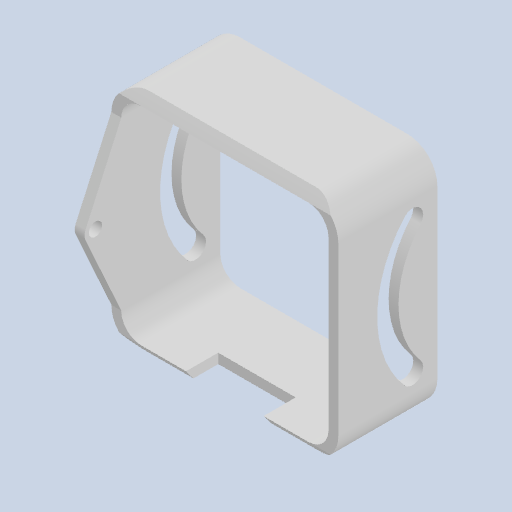
# Autodesk Inventor part: lidar_base
Saved by Autodesk Inventor 2022 (Build 260153000, 153)
## iProperties
Created: 2024-10-20
Part Number: lidar_base
Material: Типовые
Document SubType Name: Modeling
Designer: Andrey
Density: 1 g/cm^3
Appearance: По умолчанию
Author: Andrey
Autodesk Inventor part; units mm, degrees
ref_plane "YZ Plane" through (0, 0, 0) normal (1, 0, 0) x (0, 1, 0)
ref_plane "РабПлоскость1" through (-16.75, -17.4, 16.3) normal (0, 0, 1) x (1, 0, 0)
sketch "Эскиз1" plane through (0, 0, 0) normal (0, 0, 1) x (1, 0, 0)
  line L0 (-18.1779, 4.2816) -> (-18.69, 4.2816) projected
  line L1 (-18.69, 4.2816) -> (-18.69, -13.75) projected
  arc A0 (-18.69, -13.75) -> (-13.75, -18.69) centre (-13.75, -13.75) ccw projected
  line L2 (-13.75, -18.69) -> (13.75, -18.69) projected
  arc A1 (13.75, -18.69) -> (18.69, -13.75) centre (13.75, -13.75) ccw projected
  line L3 (18.69, -13.75) -> (18.69, 13.75) projected
  arc A2 (18.69, 13.75) -> (13.75, 18.69) centre (13.75, 13.75) ccw projected
  line L4 (13.75, 18.69) -> (-13.75, 18.69) projected
  arc A3 (-13.75, 18.69) -> (-18.69, 13.75) centre (-13.75, 13.75) ccw projected
  line L5 (-18.69, 13.75) -> (-18.69, 9.7184) projected
  line L6 (-18.69, 9.7184) -> (-18.1779, 9.7184) projected
  line L7 (-18.1779, 13.75) -> (-18.1779, 9.7184) projected
  arc A4 (-13.75, 18.1779) -> (-18.1779, 13.75) centre (-13.75, 13.75) ccw projected
  line L8 (13.75, 18.1779) -> (-13.75, 18.1779) projected
  arc A5 (18.1779, 13.75) -> (13.75, 18.1779) centre (13.75, 13.75) ccw projected
  line L9 (18.1779, -13.75) -> (18.1779, 13.75) projected
  arc A6 (13.75, -18.1779) -> (18.1779, -13.75) centre (13.75, -13.75) ccw projected
  line L10 (-13.75, -18.1779) -> (13.75, -18.1779) projected
  arc A7 (-18.1779, -13.75) -> (-13.75, -18.1779) centre (-13.75, -13.75) ccw projected
  line L11 (-18.1779, 4.2816) -> (-18.1779, -13.75) projected
  line L12 (-18.1779, 4.2816) -> (-18.69, 4.2816)
  line L13 (-18.69, 4.2816) -> (-18.69, 9.7184)
  line L14 (-18.69, 9.7184) -> (-18.1779, 9.7184)
  line L15 (-18.1779, 9.7184) -> (-18.1779, 4.2816)
  line L16 (-13.75, 16.45) -> (10.2, 16.45) projected
  arc A8 (-13.75, 16.45) -> (-16.75, 13.45) centre (-13.75, 13.45) ccw projected
  line L17 (-16.75, -10.2) -> (-16.75, 13.45) projected
  arc A9 (-16.75, -10.2) -> (-15.75, -11.2) centre (-15.75, -10.2) ccw projected
  line L18 (-14.1, -11.2) -> (-15.75, -11.2) projected
  arc A10 (-11.2, -14.1) -> (-14.1, -11.2) centre (-14.1, -14.1) ccw projected
  line L19 (-11.2, -14.1) -> (-11.2, -15.75) projected
  arc A11 (-11.2, -15.75) -> (-10.2, -16.75) centre (-10.2, -15.75) ccw projected
  line L20 (-6.3858, -16.75) -> (-10.2, -16.75) projected
  arc A12 (-5.9929, -17.075) -> (-6.3858, -16.75) centre (-6.3858, -17.15) ccw projected
  arc A13 (-5.9929, -17.075) -> (-5.6, -17.4) centre (-5.6, -17) ccw projected
  line L21 (-5.6, -17.4) -> (5.6, -17.4) projected
  arc A14 (5.6, -17.4) -> (5.9929, -17.075) centre (5.6, -17) ccw projected
  arc A15 (6.3858, -16.75) -> (5.9929, -17.075) centre (6.3858, -17.15) ccw projected
  line L22 (12.1982, -16.75) -> (6.3858, -16.75) projected
  arc A16 (12.1982, -16.75) -> (13.1981, -15.7356) centre (12.1982, -15.75) ccw projected
  arc A17 (15.7351, -13.198) -> (13.1981, -15.7356) centre (15.6978, -15.6978) ccw projected
  arc A18 (15.7351, -13.198) -> (16.75, -12.1982) centre (15.75, -12.1982) ccw projected
  line L23 (16.75, -12.1982) -> (16.75, 10.2) projected
  arc A19 (16.75, 10.2) -> (15.75, 11.2) centre (15.75, 10.2) ccw projected
  line L24 (14.1, 11.2) -> (15.75, 11.2) projected
  arc A20 (11.2, 14.1) -> (14.1, 11.2) centre (14.1, 14.1) ccw projected
  line L25 (11.2, 15.45) -> (11.2, 14.1) projected
  arc A21 (11.2, 15.45) -> (10.2, 16.45) centre (10.2, 15.45) ccw projected
  circle A22 centre (7, 14.5) radius 0.95 projected
  circle A23 centre (0, 14.6) radius 0.75 projected
  circle A24 centre (-7.5, -13.8) radius 0.95 projected
  circle A25 centre (-14.9, 2) radius 0.75 projected
  circle A26 centre (8.272, -2.7758) radius 0.5 projected
  circle A27 centre (8.6932, -0.0132) radius 0.5 projected
  circle A28 centre (8.2597, 2.7621) radius 0.5 projected
  circle A29 centre (-2.2984, 14.2551) radius 0.5 projected
  circle A30 centre (-4.5412, 14.2552) radius 0.5 projected
  circle A31 centre (13.75, -13.75) radius 3.5
  circle A32 centre (-13.75, -13.75) radius 3.5
  circle A33 centre (13.75, 13.75) radius 3.5
  circle A34 centre (-13.75, 13.75) radius 3.5
  line L26 (-17.25, 13.75) -> (-17.25, -13.75)
  line L27 (-13.75, -17.25) -> (13.75, -17.25)
  line L28 (17.25, -13.75) -> (17.25, 13.75)
  line L29 (13.75, 17.25) -> (-13.75, 17.25)
  arc A35 (13.75, -17.25) -> (17.25, -13.75) centre (13.75, -13.75) ccw
  arc A36 (-17.25, -13.75) -> (-13.75, -17.25) centre (-13.75, -13.75) ccw
  arc A37 (-13.75, 17.25) -> (-17.25, 13.75) centre (-13.75, 13.75) ccw
  arc A38 (17.25, 13.75) -> (13.75, 17.25) centre (13.75, 13.75) ccw
  line L30 (-13.75, 17.05) -> (13.75, 17.05)
  arc A39 (17.05, 13.75) -> (13.75, 17.05) centre (13.75, 13.75) ccw
  line L31 (17.05, 13.75) -> (17.05, -13.75)
  arc A40 (13.75, -17.05) -> (17.05, -13.75) centre (13.75, -13.75) ccw
  line L32 (13.75, -17.05) -> (-13.75, -17.05)
  arc A41 (-17.05, -13.75) -> (-13.75, -17.05) centre (-13.75, -13.75) ccw
  line L33 (-17.05, -13.75) -> (-17.05, 13.75)
  arc A42 (-13.75, 17.05) -> (-17.05, 13.75) centre (-13.75, 13.75) ccw
  line L34 (6.3858, -18.69) -> (-6.3858, -18.69)
  line L35 (-6.3858, -18.69) -> (-6.3858, -14.69)
  line L36 (-6.3858, -14.69) -> (6.3858, -14.69)
  line L37 (6.3858, -14.69) -> (6.3858, -18.69)
  point P0 (0, 0)
  point P1 (12.5838, -17.05)
  point P2 (5.9122, -17.25)
  point P3 (5.9985, -17.05)
  point P4 (-6.3858, -17.05)
  point P5 (6.3858, -17.05)
  point P6 (-6.3858, -18.69)
  dimension "d0" = 7
  dimension "d2" = 7
  dimension "d3" = 7
  dimension "d4" = 7
  dimension "d5" = 0.2
  dimension "d8" = 4
  constraints: 32 end point, 24 point on circle, 12 centre point, 12 tangent, 4 coincident, 4 parallel, 3 point on line, 2 concentric, 2 horizontal, 2 perpendicular, 7 other
  measures "d0" diameter of A31
  measures "d2" diameter of A32
  measures "d3" diameter of A33
  measures "d4" diameter of A34
  measures "d5" distance between parallel lines of L29 L30
  measures "d8" distance of L34.end L35.end
extrude "Выдавливание1" add sketch "Эскиз1" along normal up to surface (16.3 mm away) contours L11 A7 L10 L35 L2 A0 L1 L0 | L15 L7 A4 L8 A5 L9 A6 L10 L37 L27 A31 L28 A33 L29 A34 L26 A32 L35 A7 L11 | L0 L13 L6 L15 | L6 L5 A3 L4 A2 L3 A1 L2 L37 L10 A6 L9 A5 L8 A4 L7 | L27 A32 L32 L35 | L37 L32 A31 L27 | A32 L33 A41 L32 | A31 L32 A40 L31 | L26 A34 L33 A32 | A31 L31 A33 L28 | A34 L30 A42 L33 | A33 L31 A39 L30 | L29 A33 L30 A34
sketch "Эскиз2" plane through (0, 0, 0) normal (0, 0, -1) x (-1, 0, 0)
  line L0 (6.3858, -18.69) -> (6.3858, -17.05) projected
  line L1 (-6.3858, -17.05) -> (-6.3858, -18.69) projected
  line L2 (6.3858, -18.69) -> (-6.3858, -18.69)
  line L3 (-6.3858, -18.69) -> (-6.3858, -17.05)
  line L4 (-6.3858, -17.05) -> (6.3858, -17.05)
  line L5 (6.3858, -17.05) -> (6.3858, -18.69)
  point P0 (0, 0)
  constraints: 8 end point, 2 parallel, 1 horizontal, 1 perpendicular
extrude "Выдавливание2" add sketch "Эскиз2" against normal blind 11
sketch "Эскиз3" plane through (-18.69, -13.75, 0) normal (-1, 0, 0) x (0, 0, 1)
  circle A0 centre (-8.4, 13.75) radius 18.69 projected
  line L0 (0, 13.75) -> (16.3, 13.75)
  line L1 (16.3, 27.5) -> (16.3, 0) projected
  circle A1 centre (-8.4, 13.75) radius 14.8
  line L2 (0, 13.75) -> (16.3, 13.75)
  line L3 (0, 0) -> (0, 27.5) projected
  circle A2 centre (8.15, 13.75) radius 1.75
  circle A3 centre (-8.4, 13.75) radius 18.3
  circle A4 centre (4.0904, 24.6078) radius 1.75
  circle A5 centre (4.0904, 2.8922) radius 1.75
  line L4 (-8.4, 13.75) -> (22.7381, 2.4167) projected
  line L5 (-8.4, 13.75) -> (22.7381, 25.0833) projected
  line L6 (4.0904, 2.8922) -> (-8.4, 13.75)
  line L7 (-8.4, 13.75) -> (4.0904, 24.6078)
  circle A6 centre (7.5861, 18.0335) radius 1.75
  circle A7 centre (7.5861, 9.4665) radius 1.75
  line L8 (-8.4, 13.75) -> (7.5861, 18.0335)
  line L9 (7.5861, 9.4665) -> (-8.4, 13.75)
  point P0 (5.4112, 25.7559)
  point P1 (2.7697, 23.4597)
  point P2 (2.7697, 4.0403)
  point P3 (5.4112, 1.7441)
  dimension "d12" = 3.5
  dimension "d13" = 3.5
  dimension "d14" = 3.5
  dimension "d26" = 30
  dimension "d27" = 15
  dimension "d28" = 26
  dimension "d29" = 26
  constraints: 12 end point, 8 tangent, 7 centre point, 2 coincident, 2 midpoint, 1 perpendicular
  measures "d12" diameter of A2
  measures "d13" diameter of A4
  measures "d14" diameter of A5
  measures "d26" angle of L9 L8
  measures "d27" angle of L9 L0
  measures "d28" angle of L8 L7
  measures "d29" angle of L6 L9
extrude "Выдавливание3" cut sketch "Эскиз3" against normal blind 40 contours A2 L0 | L0 A2 | A3 A7 A1 A2 | A2 A1 A6 A3 | L5 A6 A1 A4 A3 | A3 A6 L5 | L4 A7 A3 | A3 A5 A1 L4 A7 | A6 L5 | A7 L4 | A4 | L5 A6 | A5 | A7 L4 | A1 L5 A6 | A7 L4 A1
sketch "Эскиз5" plane through (-18.69, -13.75, 16.3) normal (-1, 0, 0) x (0, 0, 1)
  circle A0 centre (4.2399, 13.75) radius 1.1 projected
  circle A1 centre (4.2399, 13.75) radius 1.8
  line L0 (5.8801, 13.0086) -> (0, 0)
  line L1 (0, 27.5) -> (0, 0) projected
  line L2 (5.8801, 14.4914) -> (0, 27.5)
  point P0 (-16.3, 13.75)
  dimension "d23" = 3.6
  constraints: 4 end point, 2 point on circle, 2 tangent, 1 centre point, 1 coincident
  measures "d23" diameter of A1
extrude "Выдавливание5" add sketch "Эскиз5" against normal up to surface (1.64 mm away)
sketch "Эскиз6" plane through (-18.69, -13.75, 0) normal (-1, 0, 0) x (0, 0, 1)
  circle A0 centre (-8.4, 13.75) radius 30.7399 projected
  line L0 (0, -3.3) -> (16.3, -3.3) projected
  line L1 (0, 30.8) -> (16.3, 30.8) projected
  line L2 (16.3, -3.3) -> (16.3, 0) projected
  circle A1 centre (-8.4, 13.75) radius 30.0132
  circle A2 centre (-8.4, 13.75) radius 32.0132
  line L3 (16.3, -3.3) -> (18.6951, -3.3)
  line L4 (11, -4.94) -> (16.3, -4.94) projected
  line L5 (15.0835, -4.94) -> (17.5909, -4.94)
  line L6 (0, 30.8) -> (16.3, 30.8) projected
  line L7 (16.3, 30.8) -> (18.6951, 30.8)
  line L8 (0, 32.44) -> (16.3, 32.44) projected
  line L9 (15.0835, 32.44) -> (17.5909, 32.44)
  point P0 (0, 13.75)
  point P1 (16.3, 30.8)
  dimension "d30" = 2
  constraints: 8 end point, 7 point on circle, 3 point on line, 2 centre point, 2 collinear, 1 coincident, 1 horizontal
  measures "d30" radial gap between concentric circles of A1 A2
ref_plane "РабПлоскость2" through (19.19, -20.45, 0) normal (-1, 0, 0) x (0, 0, 1)
extrude "Выдавливание6" cut sketch "Эскиз6" against normal blind 40 contours L7 A1 L8 A0 | A0 L8 L9 A2 L7 | L3 A2 L5 L4 A0 | A0 L4 A1 L3
equation "\"d27\" = 0.5 * d26"
